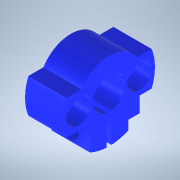
# Autodesk Inventor part: セットカラ―
Saved by Autodesk Inventor 2022.3 (Build 263350000, 350)
## iProperties
Created: 2020-01-17
Part Number: セットカラ―
Material: ABS プラスチック
Document SubType Name: Modeling
Designer: Hagihara Yuya
Density: 1.06 g/cm^3
Appearance: 青 - 壁塗料 - 光沢
Author: Hagihara Yuya
Autodesk Inventor part; units mm, degrees
ref_plane "YZ Plane" through (0, 0, 0) normal (1, 0, 0) x (0, 1, 0)
ref_plane "XZ Plane" through (0, 0, 0) normal (0, 1, 0) x (-1, 0, 0)
ref_plane "XY Plane" through (0, 0, 0) normal (0, 0, 1) x (1, 0, 0)
sketch "スケッチ1" plane through (0, 0, 0) normal (1, 0, 0) x (0, 1, 0)
  circle A0 centre (0, 0) radius 4.2
  circle A1 centre (0, 0) radius 8.5
  line L0 (0, 5) -> (-12, 5)
  line L1 (-12, 5) -> (-12, -5) construction
  line L2 (-12, -5) -> (0, -5)
  line L3 (0, -5) -> (0, 5) construction
  line L4 (-12, 0.6) -> (0, 0.6)
  line L5 (0, 0.6) -> (0, -0.6)
  line L6 (0, -0.6) -> (-12, -0.6)
  line L7 (-12, -0.6) -> (-12, 0.6)
  line L8 (4.5, 12) -> (-4.5, 12) construction
  line L9 (-4.5, 12) -> (-4.5, -12)
  line L10 (-4.5, -12) -> (4.5, -12) construction
  line L11 (4.5, -12) -> (4.5, 12)
  line L12 (4.5, 12) -> (-4.5, -12) construction
  line L13 (-4.5, 12) -> (4.5, -12) construction
  arc A2 (4.5, 11.1243) -> (-4.5, 11.1243) centre (0, 0) ccw
  arc A3 (-4.5, -11.1243) -> (4.5, -11.1243) centre (0, 0) ccw
  arc A4 (-10.9087, 5) -> (-10.9087, -5) centre (0, 0) ccw
  point P0 (-11, 3.3541)
  point P1 (-11, -3.3541)
  point P2 (-6.8739, 5)
  point P3 (-6.8739, -5)
  point P4 (-4.1569, 0.6)
  point P5 (-4.1569, -0.6)
  point P6 (-12, -0.6)
  point P7 (-8.4788, -0.6)
  point P8 (-8.4788, 0.6)
  point P9 (0, -4.2)
  point P10 (0, 4.2)
  point P11 (0, 0.6)
  point P12 (-4.5, -5)
  point P13 (4.5, -7.2111)
  point P14 (4.5, 7.2111)
  point P15 (-4.5, 5)
  point P16 (-4.5, -7.2111)
  point P17 (-4.5, 7.2111)
  point P18 (-4.5, 0.6)
  point P19 (-4.5, -0.6)
  point P20 (-11.985, 0.6)
  point P21 (-11.985, -0.6)
  dimension "d0" = 8.4
  dimension "d1" = 17
  dimension "d2" = 5
  dimension "d3" = 5
  dimension "d4" = 12
  dimension "d18" = 1.2
  dimension "d19" = 0.6
  dimension "d45" = 9
  dimension "d46" = 24
  constraints: 28 end point, 8 point on line, 6 parallel, 6 point on circle, 5 centre point, 5 coincident, 3 horizontal, 3 midpoint, 3 perpendicular, 3 tangent
  measures "d0" diameter of A0
  measures "d1" diameter of A1
  measures "d2" distance from line of L2 point (0, 0)
  measures "d3" distance from line of point (0, 0) L0
  measures "d4" distance of L1.end L2.end
  measures "d18" distance between parallel lines of L4 L6
  measures "d19" distance from line of point (0, 0) L6
  measures "d45" distance of L9.end L10.end
  measures "d46" distance of L8.end L9.end
extrude "押し出し1" add sketch "スケッチ1" along normal blind 10 contours A0 L4 L9 A1 L11 L6 | L4 A1 L0 L9 | L9 L2 A1 L6 | L4 A4 L0 A1 | A1 L2 A4 L6 | L9 A2 L11 A1 | A1 L11 A3 L9 | A1 L11
sketch "スケッチ2" plane through (10, 0, 0) normal (1, 0, 0) x (0, 0, -1)
  line L0 (16.8, 0) -> (-16.8, 0) projected
  point P0 (0, 0)
  point P1 (-8, 0)
  point P2 (8, 0)
  dimension "d7" = 8
  dimension "d8" = 8
  constraints: 2 point on line
  measures "d7" distance of point (8, 0) point (0, 0)
  measures "d8" distance of point (-8, 0) point (0, 0)
hole "穴1" at (10, 0, 8) at (10, 0, -8) direction (-1, 0, 0) diameter 3.4 end through all counterbore diameter 6.5 counterbore depth 4
sketch "スケッチ3" plane through (0, -4.5, 5) normal (0, 0, 1) x (1, 0, 0)
  line L0 (0, 0) -> (10, 0) projected
  point P0 (5, -4)
  point P1 (5, 0)
  dimension "d56" = 4
  constraints: 1 midpoint, 1 vertical alignment
  measures "d56" distance from line of point (5, -4) L0
hole "穴2" at (5, -8.5, 5) direction (0, 0, -1) diameter 4.2 end through all
sketch "スケッチ7" plane through (0, -10.9087, -5) normal (0, 0, -1) x (-1, 0, 0)
  circle A0 centre (-5, 2.4087) radius 2.1 projected
  line L0 (-7.0207, -1.0913) -> (-9.0415, 2.4087)
  line L1 (-9.0415, 2.4087) -> (-7.0207, 5.9087)
  line L2 (-7.0207, 5.9087) -> (-2.9793, 5.9087)
  line L3 (-2.9793, 5.9087) -> (-0.9585, 2.4087)
  line L4 (-0.9585, 2.4087) -> (-2.9793, -1.0913)
  line L5 (-2.9793, -1.0913) -> (-7.0207, -1.0913)
  line L6 (0, 6.4087) -> (-10, 6.4087) projected
  line L7 (-10, 0) -> (-10, 6.4087) projected
  line L8 (0, 0) -> (0, 6.4087) projected
  line L9 (-10, 2.4087) -> (-9.0415, 2.4087)
  line L10 (-0.9585, 2.4087) -> (0, 2.4087)
  circle A1 centre (-9.0415, 2.4087) radius 0.2
  circle A2 centre (-7.0207, -1.0913) radius 0.2
  circle A3 centre (-2.9793, -1.0913) radius 0.2
  circle A4 centre (-0.9585, 2.4087) radius 0.2
  circle A5 centre (-2.9793, 5.9087) radius 0.2
  circle A6 centre (-7.0207, 5.9087) radius 0.2
  point P0 (0, 10.9087)
  point P1 (-9.2415, 2.4087)
  point P2 (-8.9415, 2.5819)
  point P3 (-7.1207, 5.7355)
  point P4 (-6.8207, 5.9087)
  point P5 (-3.1793, 5.9087)
  point P6 (-2.8793, 5.7355)
  point P7 (-1.0585, 2.5819)
  point P8 (-0.7585, 2.4087)
  dimension "d48" = 7
  dimension "d49" = 0.4
  dimension "d52" = 360
  constraints: 16 end point, 6 centre point, 4 coincident, 3 horizontal alignment, 2 point on line, 30 other
  measures "d48" distance between parallel lines of L4 L1
  measures "d49" diameter of A1
extrude "押し出し5" add sketch "スケッチ7" along normal blind 3 contours L9 L7 L6 L8 L10 A4 L3 A5 L2 A6 L1 A1
equation "\"d3\" = d2"
equation "\"d19\" = 0.5 * d18"
equation "\"d8\" = d7"
